Autodesk Inventor part; units mm, degrees
(part 2 of 6)
  line L517 (-101.2642, 134.6037) -> (-101.2642, 126.9657)
  line L518 (-101.2642, 126.9657) -> (-97.138, 126.9657)
  spline S136 degree 2 poles (-97.138, 126.9657) (-96.7341, 126.9657) (-96.1722, 126.4038) (-96.1722, 126) knots 0 0 0 1 2 2 2
  spline S137 degree 2 poles (-96.1722, 126) (-96.1722, 125.6137) (-96.7341, 125.0518) (-97.138, 125.0518) knots 0 0 0 1 2 2 2
  line L519 (-97.138, 125.0518) -> (-101.2642, 125.0518)
  line L520 (-101.2642, 125.0518) -> (-101.2642, 117.4139)
  line L521 (-101.2642, 117.4139) -> (-96.1547, 117.4139)
  spline S138 degree 2 poles (-96.1547, 117.4139) (-95.7684, 117.4139) (-95.2065, 116.852) (-95.2065, 116.4482) knots 0 0 0 1 2 2 2
  spline S139 degree 2 poles (-95.2065, 116.4482) (-95.2065, 116.0794) (-95.7684, 115.5) (-96.1547, 115.5) knots 0 0 0 1 2 2 2
  line L522 (-96.1547, 115.5) -> (-102.2299, 115.5)
  spline S140 degree 2 poles (-102.2299, 115.5) (-102.6162, 115.5) (-103.1781, 116.0619) (-103.1781, 116.4482) knots 0 0 0 1 2 2 2
  line L523 (-103.1781, 116.4482) -> (-103.1781, 135.5518)
  spline S141 degree 2 poles (-65.183, 124.1564) (-64.744, 124.2793) (-64.3577, 124.648) knots 0 0 0 1 1 1
  spline S142 degree 2 poles (-64.3577, 124.648) (-63.7958, 125.2099) (-63.7958, 126) knots 0 0 0 1 1 1
  line L524 (-63.7958, 126) -> (-63.7958, 132.6898)
  spline S143 degree 2 poles (-63.7958, 132.6898) (-63.7958, 133.4799) (-64.9196, 134.6037) (-65.7097, 134.6037) knots 0 0 0 1 2 2 2
  line L525 (-65.7097, 134.6037) -> (-68.8878, 134.6037)
  line L526 (-68.8878, 134.6037) -> (-68.8878, 116.4482)
  spline S144 degree 2 poles (-68.8878, 116.4482) (-68.8878, 116.0619) (-69.4497, 115.5) (-69.8535, 115.5) knots 0 0 0 1 2 2 2
  spline S145 degree 2 poles (-69.8535, 115.5) (-70.2398, 115.5) (-70.8017, 116.0619) (-70.8017, 116.4482) knots 0 0 0 1 2 2 2
  line L527 (-70.8017, 116.4482) -> (-70.8017, 135.5518)
  spline S146 degree 2 poles (-70.8017, 135.5518) (-70.8017, 135.9557) (-70.2398, 136.5) (-69.8535, 136.5) knots 0 0 0 1 2 2 2
  line L528 (-69.8535, 136.5) -> (-65.7097, 136.5)
  spline S147 degree 2 poles (-65.7097, 136.5) (-64.1295, 136.5) (-61.882, 134.2701) (-61.882, 132.6898) knots 0 0 0 1 2 2 2
  line L529 (-61.882, 132.6898) -> (-61.882, 126)
  spline S148 degree 2 poles (-61.882, 126) (-61.882, 124.4373) (-63.0057, 123.3135) knots 0 0 0 1 1 1
  spline S149 degree 2 poles (-63.0057, 123.3135) (-63.3569, 122.9624) (-63.7432, 122.7341) knots 0 0 0 1 1 1
  line L530 (-63.7432, 122.7341) -> (-61.3552, 116.8696)
  spline S150 degree 2 poles (-61.3552, 116.8696) (-61.2499, 116.6589) (-61.2499, 116.4482) knots 0 0 0 1 1 1
  spline S151 degree 2 poles (-61.2499, 116.4482) (-61.2499, 116.3077) (-61.3025, 116.1672) knots 0 0 0 1 1 1
  spline S152 degree 2 poles (-61.3025, 116.1672) (-61.4254, 115.7809) (-61.7766, 115.6054) knots 0 0 0 1 1 1
  spline S153 degree 2 poles (-61.7766, 115.6054) (-61.9873, 115.5) (-62.198, 115.5) knots 0 0 0 1 1 1
  spline S154 degree 2 poles (-62.198, 115.5) (-62.356, 115.5) (-62.4965, 115.5351) knots 0 0 0 1 1 1
  spline S155 degree 2 poles (-62.4965, 115.5351) (-62.8828, 115.658) (-63.0584, 116.0268) knots 0 0 0 1 1 1
  line L531 (-63.0584, 116.0268) -> (-65.78, 122.7692)
  spline S156 degree 2 poles (-65.78, 122.7692) (-65.9029, 122.9799) (-65.9029, 123.2433) knots 0 0 0 1 1 1
  spline S157 degree 2 poles (-65.9029, 123.2433) (-65.9029, 123.6296) (-65.6044, 123.9281) knots 0 0 0 1 1 1
  spline S158 degree 2 poles (-65.6044, 123.9281) (-65.4288, 124.1037) (-65.183, 124.1564) knots 0 0 0 1 1 1
  spline S159 degree 2 poles (-37.0031, 134.6037) (-37.3894, 134.6037) (-37.9512, 135.148) (-37.9512, 135.5518) knots 0 0 0 1 2 2 2
  spline S160 degree 2 poles (-37.9512, 135.5518) (-37.9512, 135.9557) (-37.3894, 136.5) (-37.0031, 136.5) knots 0 0 0 1 2 2 2
  line L532 (-37.0031, 136.5) -> (-29.9972, 136.5)
  spline S161 degree 2 poles (-29.9972, 136.5) (-29.5934, 136.5) (-29.0315, 135.9557) (-29.0315, 135.5518) knots 0 0 0 1 2 2 2
  spline S162 degree 2 poles (-29.0315, 135.5518) (-29.0315, 135.148) (-29.5934, 134.6037) (-29.9972, 134.6037) knots 0 0 0 1 2 2 2
  line L533 (-29.9972, 134.6037) -> (-32.5432, 134.6037)
  line L534 (-32.5432, 134.6037) -> (-32.5432, 116.4482)
  spline S163 degree 2 poles (-32.5432, 116.4482) (-32.5432, 116.0619) (-33.0875, 115.5) (-33.4914, 115.5) knots 0 0 0 1 2 2 2
  spline S164 degree 2 poles (-33.4914, 115.5) (-33.8952, 115.5) (-34.4571, 116.0619) (-34.4571, 116.4482) knots 0 0 0 1 2 2 2
  line L535 (-34.4571, 116.4482) -> (-34.4571, 134.6037)
  line L536 (-34.4571, 134.6037) -> (-37.0031, 134.6037)
  spline S165 degree 2 poles (-4.4511, 135.8503) (-4.4511, 136.2542) (-3.8892, 136.8161) (-3.5029, 136.8161) knots 0 0 0 1 2 2 2
  spline S166 degree 2 poles (-3.5029, 136.8161) (-3.0991, 136.8161) (-2.5372, 136.2542) (-2.5372, 135.8503) knots 0 0 0 1 2 2 2
  line L537 (-2.5372, 135.8503) -> (-2.5372, 119.9599)
  spline S167 degree 2 poles (-2.5372, 119.9599) (-2.5372, 118.9064) (-1.0447, 117.4139) (0.0088, 117.4139) knots 0 0 0 1 2 2 2
  spline S168 degree 2 poles (0.0088, 117.4139) (1.0623, 117.4139) (2.5548, 118.9064) (2.5548, 119.9599) knots 0 0 0 1 2 2 2
  line L538 (2.5548, 119.9599) -> (2.5548, 135.8503)
  spline S169 degree 2 poles (2.5548, 135.8503) (2.5548, 136.2542) (3.0991, 136.8161) (3.5029, 136.8161) knots 0 0 0 1 2 2 2
  spline S170 degree 2 poles (3.5029, 136.8161) (3.9068, 136.8161) (4.4686, 136.2542) (4.4686, 135.8503) knots 0 0 0 1 2 2 2
  line L539 (4.4686, 135.8503) -> (4.4686, 119.9599)
  spline S171 degree 2 poles (4.4686, 119.9599) (4.4686, 118.1162) (1.8524, 115.5) (0.0088, 115.5) knots 0 0 0 1 2 2 2
  spline S172 degree 2 poles (0.0088, 115.5) (-1.8349, 115.5) (-4.4511, 118.1162) (-4.4511, 119.9599) knots 0 0 0 1 2 2 2
  line L540 (-4.4511, 119.9599) -> (-4.4511, 135.8503)
  spline S173 degree 2 poles (38.118, 119.9423) (38.118, 118.0987) (36.8011, 116.7993) knots 0 0 0 1 1 1
  spline S174 degree 2 poles (36.8011, 116.7993) (35.6423, 115.6054) (34.0445, 115.5) knots 0 0 0 1 1 1
  spline S175 degree 2 poles (34.0445, 115.5) (33.5704, 115.5) (33.0261, 116.0619) (33.0261, 116.4482) knots 0 0 0 1 2 2 2
  spline S176 degree 2 poles (33.0261, 116.4482) (33.0261, 116.852) (33.307, 117.1329) knots 0 0 0 1 1 1
  spline S177 degree 2 poles (33.307, 117.1329) (33.5353, 117.3788) (33.8864, 117.4139) knots 0 0 0 1 1 1
  spline S178 degree 2 poles (33.8864, 117.4139) (34.7995, 117.4841) (35.4491, 118.1513) knots 0 0 0 1 1 1
  spline S179 degree 2 poles (35.4491, 118.1513) (36.2042, 118.8888) (36.2042, 119.9423) knots 0 0 0 1 1 1
  line L541 (36.2042, 119.9423) -> (36.2042, 122.5585)
  spline S180 degree 2 poles (36.2042, 122.5585) (36.2042, 123.5945) (35.4491, 124.3495) knots 0 0 0 1 1 1
  spline S181 degree 2 poles (35.4491, 124.3495) (34.8521, 124.964) (34.0445, 125.0694) knots 0 0 0 1 1 1
  spline S182 degree 2 poles (34.0445, 125.0694) (33.5704, 125.0694) (33.307, 125.3503) knots 0 0 0 1 1 1
  spline S183 degree 2 poles (33.307, 125.3503) (33.0261, 125.6313) (33.0261, 126.0176) knots 0 0 0 1 1 1
  line L542 (33.0261, 126.0176) -> (33.0261, 126.0351)
  spline S184 degree 2 poles (33.0261, 126.0351) (33.0261, 126.439) (33.307, 126.7199) knots 0 0 0 1 1 1
  spline S185 degree 2 poles (33.307, 126.7199) (33.5704, 127.0008) (34.0445, 127.0008) knots 0 0 0 1 1 1
  spline S186 degree 2 poles (34.0445, 127.0008) (34.8521, 127.1062) (35.4491, 127.7032) knots 0 0 0 1 1 1
  spline S187 degree 2 poles (35.4491, 127.7032) (36.2042, 128.4582) (36.2042, 129.5117) knots 0 0 0 1 1 1
  line L543 (36.2042, 129.5117) -> (36.2042, 132.0928)
  spline S188 degree 2 poles (36.2042, 132.0928) (36.2042, 133.1288) (35.4491, 133.8838) knots 0 0 0 1 1 1
  spline S189 degree 2 poles (35.4491, 133.8838) (34.7995, 134.5334) (33.8864, 134.6212) knots 0 0 0 1 1 1
  spline S190 degree 2 poles (33.8864, 134.6212) (33.5353, 134.6564) (33.307, 134.9022) knots 0 0 0 1 1 1
  spline S191 degree 2 poles (33.307, 134.9022) (33.0261, 135.1656) (33.0261, 135.5694) knots 0 0 0 1 1 1
  spline S192 degree 2 poles (33.0261, 135.5694) (33.0261, 135.9732) (33.5704, 136.5176) (34.0445, 136.5176) knots 0 0 0 1 2 2 2
  spline S193 degree 2 poles (34.0445, 136.5176) (35.6423, 136.4122) (36.8011, 135.2358) knots 0 0 0 1 1 1
  spline S194 degree 2 poles (36.8011, 135.2358) (38.118, 133.9365) (38.118, 132.0928) knots 0 0 0 1 1 1
  line L544 (38.118, 132.0928) -> (38.118, 129.5117)
  spline S195 degree 2 poles (38.118, 129.5117) (38.118, 127.3344) (36.45, 126.0176) knots 0 0 0 1 1 1
  spline S196 degree 2 poles (36.45, 126.0176) (38.118, 124.7182) (38.118, 122.5585) knots 0 0 0 1 1 1
  line L545 (38.118, 122.5585) -> (38.118, 119.9423)
  spline S197 degree 2 poles (29.1983, 135.5694) (29.1983, 135.9732) (29.7602, 136.5176) (30.1465, 136.5176) knots 0 0 0 1 2 2 2
  spline S198 degree 2 poles (30.1465, 136.5176) (30.5503, 136.5176) (31.1122, 135.9732) (31.1122, 135.5694) knots 0 0 0 1 2 2 2
  line L546 (31.1122, 135.5694) -> (31.1122, 116.4657)
  spline S199 degree 2 poles (31.1122, 116.4657) (31.1122, 116.0794) (30.5503, 115.5176) (30.1465, 115.5176) knots 0 0 0 1 2 2 2
  spline S200 degree 2 poles (30.1465, 115.5176) (29.7602, 115.5176) (29.1983, 116.0794) (29.1983, 116.4657) knots 0 0 0 1 2 2 2
  line L547 (29.1983, 116.4657) -> (29.1983, 135.5694)
  spline S201 degree 2 poles (69.8448, 126.9657) (70.2486, 126.9657) (70.8105, 126.4038) (70.8105, 126) knots 0 0 0 1 2 2 2
  spline S202 degree 2 poles (70.8105, 126) (70.8105, 125.6137) (70.2486, 125.0518) (69.8448, 125.0518) knots 0 0 0 1 2 2 2
  line L548 (69.8448, 125.0518) -> (65.7185, 125.0518)
  line L549 (65.7185, 125.0518) -> (65.7185, 116.4482)
  spline S203 degree 2 poles (65.7185, 116.4482) (65.7185, 116.0619) (65.1566, 115.5) (64.7528, 115.5) knots 0 0 0 1 2 2 2
  spline S204 degree 2 poles (64.7528, 115.5) (64.3665, 115.5) (63.8046, 116.0619) (63.8046, 116.4482) knots 0 0 0 1 2 2 2
  line L550 (63.8046, 116.4482) -> (63.8046, 135.5518)
  spline S205 degree 2 poles (63.8046, 135.5518) (63.8046, 135.9557) (64.3665, 136.5) (64.7528, 136.5) knots 0 0 0 1 2 2 2
  line L551 (64.7528, 136.5) -> (70.828, 136.5)
  spline S206 degree 2 poles (70.828, 136.5) (71.2143, 136.5) (71.7762, 135.9557) (71.7762, 135.5518) knots 0 0 0 1 2 2 2
  spline S207 degree 2 poles (71.7762, 135.5518) (71.7762, 135.1656) (71.2143, 134.6037) (70.828, 134.6037) knots 0 0 0 1 2 2 2
  line L552 (70.828, 134.6037) -> (65.7185, 134.6037)
  line L553 (65.7185, 134.6037) -> (65.7185, 126.9657)
  line L554 (65.7185, 126.9657) -> (69.8448, 126.9657)
  spline S208 degree 2 poles (96.2249, 134.6037) (95.8211, 134.6037) (95.2592, 135.148) (95.2592, 135.5518) knots 0 0 0 1 2 2 2
  spline S209 degree 2 poles (95.2592, 135.5518) (95.2592, 135.9557) (95.8211, 136.5) (96.2249, 136.5) knots 0 0 0 1 2 2 2
  line L555 (96.2249, 136.5) -> (103.5468, 136.5)
  spline S210 degree 2 poles (103.5468, 136.5) (103.9331, 136.5) (104.495, 135.9557) (104.495, 135.5518) knots 0 0 0 1 2 2 2
  spline S211 degree 2 poles (104.495, 135.5518) (104.495, 135.3587) (104.4247, 135.1831) knots 0 0 0 1 1 1
  line L556 (104.4247, 135.1831) -> (97.612, 117.4139)
  line L557 (97.612, 117.4139) -> (103.5468, 117.4139)
  spline S212 degree 2 poles (103.5468, 117.4139) (103.9331, 117.4139) (104.495, 116.852) (104.495, 116.4482) knots 0 0 0 1 2 2 2
  spline S213 degree 2 poles (104.495, 116.4482) (104.495, 116.0794) (103.9331, 115.5) (103.5468, 115.5) knots 0 0 0 1 2 2 2
  line L558 (103.5468, 115.5) -> (96.2249, 115.5)
  spline S214 degree 2 poles (96.2249, 115.5) (95.8386, 115.5) (95.2768, 116.0794) (95.2768, 116.4482) knots 0 0 0 1 2 2 2
  spline S215 degree 2 poles (95.2768, 116.4482) (95.2768, 116.694) (95.3645, 116.8871) knots 0 0 0 1 1 1
  line L559 (95.3645, 116.8871) -> (102.1421, 134.6037)
  line L560 (102.1421, 134.6037) -> (96.2249, 134.6037)
  spline S216 degree 2 poles (133.3421, 121.8211) (133.7284, 121.8211) (134.2903, 121.2592) (134.2903, 120.8554) knots 0 0 0 1 2 2 2
  spline S217 degree 2 poles (134.2903, 120.8554) (134.2903, 120.4691) (133.7284, 119.9072) (133.3421, 119.9072) knots 0 0 0 1 2 2 2
  line L561 (133.3421, 119.9072) -> (130.164, 119.9072)
  line L562 (130.164, 119.9072) -> (129.1983, 116.2901)
  spline S218 degree 2 poles (129.1983, 116.2901) (129.1105, 115.9916) (128.9174, 115.7809) knots 0 0 0 1 1 1
  spline S219 degree 2 poles (128.9174, 115.7809) (128.6364, 115.5) (128.2501, 115.5) knots 0 0 0 1 1 1
  spline S220 degree 2 poles (128.2501, 115.5) (127.8463, 115.5) (127.2844, 116.0619) (127.2844, 116.4482) knots 0 0 0 1 2 2 2
  spline S221 degree 2 poles (127.2844, 116.4482) (127.2844, 116.5711) (127.302, 116.6589) knots 0 0 0 1 1 1
  line L563 (127.302, 116.6589) -> (132.394, 135.6572)
  spline S222 degree 2 poles (132.394, 135.6572) (132.4642, 135.9732) (132.6749, 136.2015) knots 0 0 0 1 1 1
  spline S223 degree 2 poles (132.6749, 136.2015) (132.9558, 136.5) (133.3421, 136.5) knots 0 0 0 1 1 1
  spline S224 degree 2 poles (133.3421, 136.5) (133.7284, 136.5) (134.0269, 136.2015) knots 0 0 0 1 1 1
  spline S225 degree 2 poles (134.0269, 136.2015) (134.2025, 135.9732) (134.2727, 135.6572) knots 0 0 0 1 1 1
  line L564 (134.2727, 135.6572) -> (139.3647, 116.6589)
  spline S226 degree 2 poles (139.3647, 116.6589) (139.3822, 116.5711) (139.3822, 116.4482) knots 0 0 0 1 1 1
  spline S227 degree 2 poles (139.3822, 116.4482) (139.3822, 116.0619) (138.8204, 115.5) (138.4341, 115.5) knots 0 0 0 1 2 2 2
  spline S228 degree 2 poles (138.4341, 115.5) (138.0302, 115.5) (137.7669, 115.7809) knots 0 0 0 1 1 1
  spline S229 degree 2 poles (137.7669, 115.7809) (137.5562, 115.9916) (137.4684, 116.2901) knots 0 0 0 1 1 1
  line L565 (137.4684, 116.2901) -> (133.3421, 131.7943)
  line L566 (133.3421, 131.7943) -> (130.6732, 121.8211)
  line L567 (130.6732, 121.8211) -> (133.3421, 121.8211)
  spline S230 degree 2 poles (131.0244, 141.6095) (131.5511, 141.6095) (132.3062, 140.8545) (132.3062, 140.3278) knots 0 0 0 1 2 2 2
  spline S231 degree 2 poles (132.3062, 140.3278) (132.3062, 139.801) (131.5511, 139.0635) (131.0244, 139.0635) knots 0 0 0 1 2 2 2
  spline S232 degree 2 poles (131.0244, 139.0635) (130.4976, 139.0635) (129.7602, 139.801) (129.7602, 140.3278) knots 0 0 0 1 2 2 2
  spline S233 degree 2 poles (129.7602, 140.3278) (129.7602, 140.8545) (130.4976, 141.6095) (131.0244, 141.6095) knots 0 0 0 1 2 2 2
  spline S234 degree 2 poles (135.6598, 141.6095) (136.1866, 141.6095) (136.9241, 140.8545) (136.9241, 140.3278) knots 0 0 0 1 2 2 2
  spline S235 degree 2 poles (136.9241, 140.3278) (136.9241, 139.801) (136.1866, 139.0635) (135.6598, 139.0635) knots 0 0 0 1 2 2 2
  spline S236 degree 2 poles (135.6598, 139.0635) (135.1331, 139.0635) (134.3781, 139.801) (134.3781, 140.3278) knots 0 0 0 1 2 2 2
  spline S237 degree 2 poles (134.3781, 140.3278) (134.3781, 140.8545) (135.1331, 141.6095) (135.6598, 141.6095) knots 0 0 0 1 2 2 2
  spline S238 degree 2 poles (166.6754, 121.8211) (167.0617, 121.8211) (167.6236, 121.2592) (167.6236, 120.8554) knots 0 0 0 1 2 2 2
  spline S239 degree 2 poles (167.6236, 120.8554) (167.6236, 120.4691) (167.0617, 119.9072) (166.6754, 119.9072) knots 0 0 0 1 2 2 2
  line L568 (166.6754, 119.9072) -> (163.4974, 119.9072)
  line L569 (163.4974, 119.9072) -> (162.5316, 116.2901)
  spline S240 degree 2 poles (162.5316, 116.2901) (162.4438, 115.9916) (162.2507, 115.7809) knots 0 0 0 1 1 1
  spline S241 degree 2 poles (162.2507, 115.7809) (161.9698, 115.5) (161.5835, 115.5) knots 0 0 0 1 1 1
  spline S242 degree 2 poles (161.5835, 115.5) (161.1796, 115.5) (160.6178, 116.0619) (160.6178, 116.4482) knots 0 0 0 1 2 2 2
  spline S243 degree 2 poles (160.6178, 116.4482) (160.6178, 116.5711) (160.6353, 116.6589) knots 0 0 0 1 1 1
  line L570 (160.6353, 116.6589) -> (165.7273, 135.6572)
  spline S244 degree 2 poles (165.7273, 135.6572) (165.7975, 135.9732) (166.0082, 136.2015) knots 0 0 0 1 1 1
  spline S245 degree 2 poles (166.0082, 136.2015) (166.2892, 136.5) (166.6754, 136.5) knots 0 0 0 1 1 1
  spline S246 degree 2 poles (166.6754, 136.5) (167.0617, 136.5) (167.3602, 136.2015) knots 0 0 0 1 1 1
  spline S247 degree 2 poles (167.3602, 136.2015) (167.5358, 135.9732) (167.606, 135.6572) knots 0 0 0 1 1 1
  line L571 (167.606, 135.6572) -> (172.698, 116.6589)
  spline S248 degree 2 poles (172.698, 116.6589) (172.7156, 116.5711) (172.7156, 116.4482) knots 0 0 0 1 1 1
  spline S249 degree 2 poles (172.7156, 116.4482) (172.7156, 116.0619) (172.1537, 115.5) (171.7674, 115.5) knots 0 0 0 1 2 2 2
  spline S250 degree 2 poles (171.7674, 115.5) (171.3636, 115.5) (171.1002, 115.7809) knots 0 0 0 1 1 1
  spline S251 degree 2 poles (171.1002, 115.7809) (170.8895, 115.9916) (170.8017, 116.2901) knots 0 0 0 1 1 1
  line L572 (170.8017, 116.2901) -> (166.6754, 131.7943)
  line L573 (166.6754, 131.7943) -> (164.0065, 121.8211)
  line L574 (164.0065, 121.8211) -> (166.6754, 121.8211)
  spline S252 degree 2 poles (164.3577, 141.6095) (164.8845, 141.6095) (165.6395, 140.8545) (165.6395, 140.3278) knots 0 0 0 1 2 2 2
  spline S253 degree 2 poles (165.6395, 140.3278) (165.6395, 139.801) (164.8845, 139.0635) (164.3577, 139.0635) knots 0 0 0 1 2 2 2
  spline S254 degree 2 poles (164.3577, 139.0635) (163.831, 139.0635) (163.0935, 139.801) (163.0935, 140.3278) knots 0 0 0 1 2 2 2
  spline S255 degree 2 poles (163.0935, 140.3278) (163.0935, 140.8545) (163.831, 141.6095) (164.3577, 141.6095) knots 0 0 0 1 2 2 2
  spline S256 degree 2 poles (168.9932, 141.6095) (169.5199, 141.6095) (170.2574, 140.8545) (170.2574, 140.3278) knots 0 0 0 1 2 2 2
  spline S257 degree 2 poles (170.2574, 140.3278) (170.2574, 139.801) (169.5199, 139.0635) (168.9932, 139.0635) knots 0 0 0 1 2 2 2
  spline S258 degree 2 poles (168.9932, 139.0635) (168.4664, 139.0635) (167.7114, 139.801) (167.7114, 140.3278) knots 0 0 0 1 2 2 2
  spline S259 degree 2 poles (167.7114, 140.3278) (167.7114, 140.8545) (168.4664, 141.6095) (168.9932, 141.6095) knots 0 0 0 1 2 2 2
  spline S260 degree 2 poles (168.1504, 88.1564) (168.5893, 88.2793) (168.9756, 88.648) knots 0 0 0 1 1 1
  spline S261 degree 2 poles (168.9756, 88.648) (169.5375, 89.2099) (169.5375, 90) knots 0 0 0 1 1 1
  line L575 (169.5375, 90) -> (169.5375, 96.6898)
  spline S262 degree 2 poles (169.5375, 96.6898) (169.5375, 97.4799) (168.4137, 98.6037) (167.6236, 98.6037) knots 0 0 0 1 2 2 2
  line L576 (167.6236, 98.6037) -> (164.4455, 98.6037)
  line L577 (164.4455, 98.6037) -> (164.4455, 80.4482)
  spline S263 degree 2 poles (164.4455, 80.4482) (164.4455, 80.0619) (163.8836, 79.5) (163.4798, 79.5) knots 0 0 0 1 2 2 2
  spline S264 degree 2 poles (163.4798, 79.5) (163.0935, 79.5) (162.5316, 80.0619) (162.5316, 80.4482) knots 0 0 0 1 2 2 2
  line L578 (162.5316, 80.4482) -> (162.5316, 99.5518)
  spline S265 degree 2 poles (162.5316, 99.5518) (162.5316, 99.9557) (163.0935, 100.5) (163.4798, 100.5) knots 0 0 0 1 2 2 2
  line L579 (163.4798, 100.5) -> (167.6236, 100.5)
  spline S266 degree 2 poles (167.6236, 100.5) (169.2039, 100.5) (171.4514, 98.2701) (171.4514, 96.6898) knots 0 0 0 1 2 2 2
  line L580 (171.4514, 96.6898) -> (171.4514, 90)
  spline S267 degree 2 poles (171.4514, 90) (171.4514, 88.4373) (170.3276, 87.3135) knots 0 0 0 1 1 1
  spline S268 degree 2 poles (170.3276, 87.3135) (169.9764, 86.9624) (169.5902, 86.7341) knots 0 0 0 1 1 1
  line L581 (169.5902, 86.7341) -> (171.9781, 80.8696)
  spline S269 degree 2 poles (171.9781, 80.8696) (172.0835, 80.6589) (172.0835, 80.4482) knots 0 0 0 1 1 1
  spline S270 degree 2 poles (172.0835, 80.4482) (172.0835, 80.3077) (172.0308, 80.1672) knots 0 0 0 1 1 1
  spline S271 degree 2 poles (172.0308, 80.1672) (171.9079, 79.7809) (171.5567, 79.6054) knots 0 0 0 1 1 1
  spline S272 degree 2 poles (171.5567, 79.6054) (171.346, 79.5) (171.1353, 79.5) knots 0 0 0 1 1 1
  spline S273 degree 2 poles (171.1353, 79.5) (170.9773, 79.5) (170.8368, 79.5351) knots 0 0 0 1 1 1
  spline S274 degree 2 poles (170.8368, 79.5351) (170.4505, 79.658) (170.2749, 80.0268) knots 0 0 0 1 1 1
  line L582 (170.2749, 80.0268) -> (167.5534, 86.7692)
  spline S275 degree 2 poles (167.5534, 86.7692) (167.4305, 86.9799) (167.4305, 87.2433) knots 0 0 0 1 1 1
  spline S276 degree 2 poles (167.4305, 87.2433) (167.4305, 87.6296) (167.729, 87.9281) knots 0 0 0 1 1 1
  spline S277 degree 2 poles (167.729, 87.9281) (167.9045, 88.1037) (168.1504, 88.1564) knots 0 0 0 1 1 1
  spline S278 degree 2 poles (130.8664, 100.3595) (131.1122, 100.5176) (131.4282, 100.5176) knots 0 0 0 1 1 1
  spline S279 degree 2 poles (131.4282, 100.5176) (131.8145, 100.5176) (132.3764, 99.9557) (132.3764, 99.5694) knots 0 0 0 1 2 2 2
  spline S280 degree 2 poles (132.3764, 99.5694) (132.3764, 99.1656) (132.113, 98.9022) knots 0 0 0 1 1 1
  spline S281 degree 2 poles (132.113, 98.9022) (132.0252, 98.8319) (131.955, 98.7617) knots 0 0 0 1 1 1
  spline S282 degree 2 poles (131.955, 98.7617) (131.7267, 98.6212) (131.5336, 98.4281) knots 0 0 0 1 1 1
  spline S283 degree 2 poles (131.5336, 98.4281) (130.7961, 97.6731) (130.7961, 96.6196) knots 0 0 0 1 1 1
  line L583 (130.7961, 96.6196) -> (130.7961, 83.398)
  spline S284 degree 2 poles (130.7961, 83.398) (130.7961, 82.3445) (131.5336, 81.607) knots 0 0 0 1 1 1
  spline S285 degree 2 poles (131.5336, 81.607) (131.7267, 81.4139) (131.955, 81.2734) knots 0 0 0 1 1 1
  spline S286 degree 2 poles (131.955, 81.2734) (132.0252, 81.2207) (132.0955, 81.1505) knots 0 0 0 1 1 1
  spline S287 degree 2 poles (132.0955, 81.1505) (132.3764, 80.8696) (132.3764, 80.4657) knots 0 0 0 1 1 1
  spline S288 degree 2 poles (132.3764, 80.4657) (132.3764, 80.0794) (131.8145, 79.5176) (131.4282, 79.5176) knots 0 0 0 1 2 2 2
  spline S289 degree 2 poles (131.4282, 79.5176) (131.1297, 79.5176) (130.9015, 79.658) knots 0 0 0 1 1 1
  spline S290 degree 2 poles (130.9015, 79.658) (130.5152, 79.9214) (130.1816, 80.255) knots 0 0 0 1 1 1
  spline S291 degree 2 poles (130.1816, 80.255) (128.8822, 81.5543) (128.8822, 83.398) knots 0 0 0 1 1 1
  line L584 (128.8822, 83.398) -> (128.8822, 96.6196)
  spline S292 degree 2 poles (128.8822, 96.6196) (128.8822, 98.4808) (130.1816, 99.7801) knots 0 0 0 1 1 1
  spline S293 degree 2 poles (130.1816, 99.7801) (130.5152, 100.1137) (130.8664, 100.3595) knots 0 0 0 1 1 1
  spline S294 degree 2 poles (134.8346, 98.6915) (134.6941, 98.7617) (134.5712, 98.8846) knots 0 0 0 1 1 1
  spline S295 degree 2 poles (134.5712, 98.8846) (134.2903, 99.1656) (134.2903, 99.5518) knots 0 0 0 1 1 1
  spline S296 degree 2 poles (134.2903, 99.5518) (134.2903, 99.9557) (134.8521, 100.5176) (135.2384, 100.5176) knots 0 0 0 1 2 2 2
  spline S297 degree 2 poles (135.2384, 100.5176) (135.5545, 100.5176) (135.8179, 100.342) knots 0 0 0 1 1 1
  spline S298 degree 2 poles (135.8179, 100.342) (136.169, 100.0962) (136.4851, 99.7801) knots 0 0 0 1 1 1
  spline S299 degree 2 poles (136.4851, 99.7801) (137.7844, 98.4808) (137.7844, 96.6196) knots 0 0 0 1 1 1
  line L585 (137.7844, 96.6196) -> (137.7844, 83.398)
  spline S300 degree 2 poles (137.7844, 83.398) (137.7844, 81.5543) (136.4851, 80.255) knots 0 0 0 1 1 1
  spline S301 degree 2 poles (136.4851, 80.255) (136.1339, 79.9038) (135.7476, 79.6405) knots 0 0 0 1 1 1
  spline S302 degree 2 poles (135.7476, 79.6405) (135.5369, 79.5) (135.2384, 79.5) knots 0 0 0 1 1 1
  spline S303 degree 2 poles (135.2384, 79.5) (134.8521, 79.5) (134.2903, 80.0794) (134.2903, 80.4482) knots 0 0 0 1 2 2 2
  spline S304 degree 2 poles (134.2903, 80.4482) (134.2903, 80.852) (134.5712, 81.1329) knots 0 0 0 1 1 1
  spline S305 degree 2 poles (134.5712, 81.1329) (134.6414, 81.2032) (134.7117, 81.2559) knots 0 0 0 1 1 1
  spline S306 degree 2 poles (134.7117, 81.2559) (134.9224, 81.3963) (135.1331, 81.607) knots 0 0 0 1 1 1
  spline S307 degree 2 poles (135.1331, 81.607) (135.8881, 82.3445) (135.8881, 83.398) knots 0 0 0 1 1 1
  line L586 (135.8881, 83.398) -> (135.8881, 96.6196)
  spline S308 degree 2 poles (135.8881, 96.6196) (135.8881, 97.6731) (135.1331, 98.4281) knots 0 0 0 1 1 1
  spline S309 degree 2 poles (135.1331, 98.4281) (134.9926, 98.5686) (134.8346, 98.6915) knots 0 0 0 1 1 1
  spline S310 degree 2 poles (93.9686, 99.3411) (93.9511, 99.4465) (93.9511, 99.5518) knots 0 0 0 1 1 1
  spline S311 degree 2 poles (93.9511, 99.5518) (93.9511, 99.9557) (94.513, 100.5) (94.9168, 100.5) knots 0 0 0 1 2 2 2
  spline S312 degree 2 poles (94.9168, 100.5) (95.3031, 100.5) (95.584, 100.2366) knots 0 0 0 1 1 1
  spline S313 degree 2 poles (95.584, 100.2366) (95.7947, 100.0084) (95.865, 99.7099) knots 0 0 0 1 1 1
  line L587 (95.865, 99.7099) -> (100.0088, 84.1881)
  line L588 (100.0088, 84.1881) -> (104.135, 99.7099)
  spline S314 degree 2 poles (104.135, 99.7099) (104.2053, 100.0084) (104.4335, 100.2366) knots 0 0 0 1 1 1
  spline S315 degree 2 poles (104.4335, 100.2366) (104.6969, 100.5) (105.1008, 100.5) knots 0 0 0 1 1 1
  spline S316 degree 2 poles (105.1008, 100.5) (105.487, 100.5) (106.0489, 99.9557) (106.0489, 99.5518) knots 0 0 0 1 2 2 2
  spline S317 degree 2 poles (106.0489, 99.5518) (106.0489, 99.4465) (106.0314, 99.3411) knots 0 0 0 1 1 1
  line L589 (106.0314, 99.3411) -> (100.9394, 80.3253)
  spline S318 degree 2 poles (100.9394, 80.3253) (100.8691, 80.0268) (100.6936, 79.7809) knots 0 0 0 1 1 1
  spline S319 degree 2 poles (100.6936, 79.7809) (100.3951, 79.5) (100.0088, 79.5) knots 0 0 0 1 1 1
  spline S320 degree 2 poles (100.0088, 79.5) (99.6225, 79.5) (99.3416, 79.7809) knots 0 0 0 1 1 1
  spline S321 degree 2 poles (99.3416, 79.7809) (99.1309, 80.0268) (99.0606, 80.3253) knots 0 0 0 1 1 1
  line L590 (99.0606, 80.3253) -> (93.9686, 99.3411)
  spline S322 degree 2 poles (65.7097, 99.5518) (65.7097, 99.9557) (66.2716, 100.5) (66.6579, 100.5) knots 0 0 0 1 2 2 2
  spline S323 degree 2 poles (66.6579, 100.5) (67.0617, 100.5) (67.6236, 99.9557) (67.6236, 99.5518) knots 0 0 0 1 2 2 2
  line L591 (67.6236, 99.5518) -> (67.6236, 80.4482)
  spline S324 degree 2 poles (67.6236, 80.4482) (67.6236, 80.0619) (67.0617, 79.5) (66.6579, 79.5) knots 0 0 0 1 2 2 2
  spline S325 degree 2 poles (66.6579, 79.5) (66.2716, 79.5) (65.7097, 80.0619) (65.7097, 80.4482) knots 0 0 0 1 2 2 2
  line L592 (65.7097, 80.4482) -> (65.7097, 99.5518)
  spline S326 degree 2 poles (29.7865, 80.9749) (29.488, 81.3261) (29.488, 81.7299) knots 0 0 0 1 1 1
  spline S327 degree 2 poles (29.488, 81.7299) (29.5231, 82.1338) (29.8041, 82.3972) knots 0 0 0 1 1 1
  spline S328 degree 2 poles (29.8041, 82.3972) (30.0674, 82.643) (30.4889, 82.643) knots 0 0 0 1 1 1
  spline S329 degree 2 poles (30.4889, 82.643) (30.8751, 82.6079) (31.2088, 82.2742) knots 0 0 0 1 1 1
  spline S330 degree 2 poles (31.2088, 82.2742) (31.9111, 81.4841) (32.9646, 81.4314) knots 0 0 0 1 1 1
  line L593 (32.9646, 81.4314) -> (33.0875, 81.4314)
  spline S331 degree 2 poles (33.0875, 81.4314) (34.0708, 81.4314) (34.7907, 82.0987) knots 0 0 0 1 1 1
  spline S332 degree 2 poles (34.7907, 82.0987) (35.5808, 82.801) (35.6335, 83.837) knots 0 0 0 1 1 1
  line L594 (35.6335, 83.837) -> (35.6335, 84.0477)
  spline S333 degree 2 poles (35.6335, 84.0477) (35.6335, 86.6814) (32.4378, 90.2107) knots 0 0 0 1 1 1
  spline S334 degree 2 poles (32.4378, 90.2107) (29.2598, 93.7224) (29.2598, 96.6722) knots 0 0 0 1 1 1
  line L595 (29.2598, 96.6722) -> (29.2598, 96.9356)
  spline S335 degree 2 poles (29.2598, 96.9356) (29.3651, 98.7968) (30.7347, 100.0259) knots 0 0 0 1 1 1
  spline S336 degree 2 poles (30.7347, 100.0259) (32.0164, 101.1672) (33.6845, 101.1672) knots 0 0 0 1 1 1
  line L596 (33.6845, 101.1672) -> (33.9479, 101.1672)
  spline S337 degree 2 poles (33.9479, 101.1672) (35.8091, 101.0619) (37.0206, 99.6923) knots 0 0 0 1 1 1
  spline S338 degree 2 poles (37.0206, 99.6923) (37.3367, 99.3411) (37.3367, 98.9548) knots 0 0 0 1 1 1
  spline S339 degree 2 poles (37.3367, 98.9548) (37.3016, 98.551) (37.0031, 98.2876) knots 0 0 0 1 1 1
  spline S340 degree 2 poles (37.0031, 98.2876) (36.7397, 98.0418) (36.371, 98.0418) knots 0 0 0 1 1 1
  spline S341 degree 2 poles (36.371, 98.0418) (35.932, 98.0594) (35.6335, 98.4105) knots 0 0 0 1 1 1
  spline S342 degree 2 poles (35.6335, 98.4105) (34.896, 99.1831) (33.8425, 99.2358) knots 0 0 0 1 1 1
  line L597 (33.8425, 99.2358) -> (33.6669, 99.2358)
  spline S343 degree 2 poles (33.6669, 99.2358) (32.7363, 99.2358) (32.0164, 98.6037) knots 0 0 0 1 1 1
  spline S344 degree 2 poles (32.0164, 98.6037) (31.2263, 97.8838) (31.1736, 96.8303) knots 0 0 0 1 1 1
  line L598 (31.1736, 96.8303) -> (31.1736, 96.6898)
  spline S345 degree 2 poles (31.1736, 96.6898) (31.1736, 94.4774) (34.4044, 90.9306) knots 0 0 0 1 1 1
  spline S346 degree 2 poles (34.4044, 90.9306) (37.5649, 87.4189) (37.5649, 84.1003) knots 0 0 0 1 1 1
  spline S347 degree 2 poles (37.5649, 84.1003) (37.5649, 83.9247) (37.5474, 83.7492) knots 0 0 0 1 1 1
  spline S348 degree 2 poles (37.5474, 83.7492) (37.442, 81.888) (36.0725, 80.6413) knots 0 0 0 1 1 1
  spline S349 degree 2 poles (36.0725, 80.6413) (34.7907, 79.5) (33.1051, 79.5) knots 0 0 0 1 1 1
  line L599 (33.1051, 79.5) -> (32.8593, 79.5)
  spline S350 degree 2 poles (32.8593, 79.5) (31.0156, 79.6054) (29.7865, 80.9749) knots 0 0 0 1 1 1
  spline S351 degree 2 poles (3.1957, 99.4816) (3.459, 99.1831) (3.459, 98.8144) knots 0 0 0 1 1 1
  spline S352 degree 2 poles (3.459, 98.8144) (3.459, 98.4105) (2.8972, 97.8487) (2.5109, 97.8487) knots 0 0 0 1 2 2 2
  spline S353 degree 2 poles (2.5109, 97.8487) (2.107, 97.8487) (1.8436, 98.1296) knots 0 0 0 1 1 1
  spline S354 degree 2 poles (1.8436, 98.1296) (1.036, 98.9197) (0, 98.9197) knots 0 0 0 1 1 1
  spline S355 degree 2 poles (0, 98.9197) (-1.0711, 98.9197) (-2.546, 97.4273) (-2.546, 96.3737) knots 0 0 0 1 2 2 2
  line L600 (-2.546, 96.3737) -> (-2.546, 83.9599)
  spline S356 degree 2 poles (-2.546, 83.9599) (-2.546, 82.9064) (-1.0711, 81.4139) (0, 81.4139) knots 0 0 0 1 2 2 2
  line L601 (0, 81.4139) -> (2.546, 81.4139)
  line L602 (2.546, 81.4139) -> (2.546, 88.7358)
  line L603 (2.546, 88.7358) -> (1.5803, 88.7358)
  spline S357 degree 2 poles (1.5803, 88.7358) (1.194, 88.7358) (0.6321, 89.2977) (0.6321, 89.6839) knots 0 0 0 1 2 2 2
  spline S358 degree 2 poles (0.6321, 89.6839) (0.6321, 90.0878) (1.194, 90.6497) (1.5803, 90.6497) knots 0 0 0 1 2 2 2
  line L604 (1.5803, 90.6497) -> (3.5117, 90.6497)
  spline S359 degree 2 poles (3.5117, 90.6497) (3.9156, 90.6497) (4.4423, 90.0878) (4.4423, 89.6839) knots 0 0 0 1 2 2 2
  line L605 (4.4423, 89.6839) -> (4.4423, 80.4482)
  spline S360 degree 2 poles (4.4423, 80.4482) (4.4423, 80.0794) (3.898, 79.5) (3.4941, 79.5) knots 0 0 0 1 2 2 2
  line L606 (3.4941, 79.5) -> (0, 79.5)
  spline S361 degree 2 poles (0, 79.5) (-1.8612, 79.5) (-4.4599, 82.0987) (-4.4599, 83.9423) knots 0 0 0 1 2 2 2
  line L607 (-4.4599, 83.9423) -> (-4.4599, 96.3913)
  spline S362 degree 2 poles (-4.4599, 96.3913) (-4.4599, 98.2349) (-1.8612, 100.8512) (0, 100.8512) knots 0 0 0 1 2 2 2
  spline S363 degree 2 poles (0, 100.8512) (1.8436, 100.8512) (3.1957, 99.4816) knots 0 0 0 1 1 1
  spline S364 degree 2 poles (-37.1084, 98.6037) (-37.5123, 98.6037) (-38.0741, 99.148) (-38.0741, 99.5518) knots 0 0 0 1 2 2 2
  spline S365 degree 2 poles (-38.0741, 99.5518) (-38.0741, 99.9557) (-37.5123, 100.5) (-37.1084, 100.5) knots 0 0 0 1 2 2 2
  line L608 (-37.1084, 100.5) -> (-29.7865, 100.5)
  spline S366 degree 2 poles (-29.7865, 100.5) (-29.4002, 100.5) (-28.8384, 99.9557) (-28.8384, 99.5518) knots 0 0 0 1 2 2 2
  spline S367 degree 2 poles (-28.8384, 99.5518) (-28.8384, 99.3587) (-28.9086, 99.1831) knots 0 0 0 1 1 1
  line L609 (-28.9086, 99.1831) -> (-35.7213, 81.4139)
  line L610 (-35.7213, 81.4139) -> (-29.7865, 81.4139)
  spline S368 degree 2 poles (-29.7865, 81.4139) (-29.4002, 81.4139) (-28.8384, 80.852) (-28.8384, 80.4482) knots 0 0 0 1 2 2 2
  spline S369 degree 2 poles (-28.8384, 80.4482) (-28.8384, 80.0794) (-29.4002, 79.5) (-29.7865, 79.5) knots 0 0 0 1 2 2 2
  line L611 (-29.7865, 79.5) -> (-37.1084, 79.5)
  spline S370 degree 2 poles (-37.1084, 79.5) (-37.4947, 79.5) (-38.0566, 80.0794) (-38.0566, 80.4482) knots 0 0 0 1 2 2 2
  spline S371 degree 2 poles (-38.0566, 80.4482) (-38.0566, 80.694) (-37.9688, 80.8871) knots 0 0 0 1 1 1
  line L612 (-37.9688, 80.8871) -> (-31.1912, 98.6037)
  line L613 (-31.1912, 98.6037) -> (-37.1084, 98.6037)
  spline S372 degree 2 poles (-70.1608, 80.4482) (-70.1608, 80.0619) (-70.7227, 79.5) (-71.1265, 79.5) knots 0 0 0 1 2 2 2
  spline S373 degree 2 poles (-71.1265, 79.5) (-71.5128, 79.5) (-72.0747, 80.0619) (-72.0747, 80.4482) knots 0 0 0 1 2 2 2
  line L614 (-72.0747, 80.4482) -> (-72.0747, 99.5694)
  spline S374 degree 2 poles (-72.0747, 99.5694) (-72.0747, 99.9732) (-71.5128, 100.5176) (-71.1265, 100.5176) knots 0 0 0 1 2 2 2
  spline S375 degree 2 poles (-71.1265, 100.5176) (-70.7227, 100.5176) (-70.4417, 100.2542) knots 0 0 0 1 1 1
  spline S376 degree 2 poles (-70.4417, 100.2542) (-70.3364, 100.1488) (-70.2837, 100.0259) knots 0 0 0 1 1 1
  line L615 (-70.2837, 100.0259) -> (-63.155, 84.7324)
  line L616 (-63.155, 84.7324) -> (-63.155, 99.5694)
  spline S377 degree 2 poles (-63.155, 99.5694) (-63.155, 99.9732) (-62.6106, 100.5176) (-62.2068, 100.5176) knots 0 0 0 1 2 2 2
  spline S378 degree 2 poles (-62.2068, 100.5176) (-61.803, 100.5176) (-61.2586, 99.9732) (-61.2586, 99.5694) knots 0 0 0 1 2 2 2
  line L617 (-61.2586, 99.5694) -> (-61.2586, 80.4306)
  spline S379 degree 2 poles (-61.2586, 80.4306) (-61.2586, 80.0619) (-61.522, 79.7809) knots 0 0 0 1 1 1
  spline S380 degree 2 poles (-61.522, 79.7809) (-61.803, 79.5) (-62.2068, 79.5) knots 0 0 0 1 1 1
  spline S381 degree 2 poles (-62.2068, 79.5) (-62.6106, 79.5) (-62.874, 79.7809) knots 0 0 0 1 1 1
  spline S382 degree 2 poles (-62.874, 79.7809) (-63.0145, 79.9214) (-63.1198, 80.1321) knots 0 0 0 1 1 1
  line L618 (-63.1198, 80.1321) -> (-70.1608, 95.3729)
  line L619 (-70.1608, 95.3729) -> (-70.1608, 80.4482)
  spline S383 degree 2 poles (-99.9912, 85.8211) (-99.6049, 85.8211) (-99.0431, 85.2592) (-99.0431, 84.8554) knots 0 0 0 1 2 2 2
  spline S384 degree 2 poles (-99.0431, 84.8554) (-99.0431, 84.4691) (-99.6049, 83.9072) (-99.9912, 83.9072) knots 0 0 0 1 2 2 2
  line L620 (-99.9912, 83.9072) -> (-103.1693, 83.9072)
  line L621 (-103.1693, 83.9072) -> (-104.135, 80.2901)
  spline S385 degree 2 poles (-104.135, 80.2901) (-104.2228, 79.9916) (-104.416, 79.7809) knots 0 0 0 1 1 1
  spline S386 degree 2 poles (-104.416, 79.7809) (-104.6969, 79.5) (-105.0832, 79.5) knots 0 0 0 1 1 1
  spline S387 degree 2 poles (-105.0832, 79.5) (-105.487, 79.5) (-106.0489, 80.0619) (-106.0489, 80.4482) knots 0 0 0 1 2 2 2
  spline S388 degree 2 poles (-106.0489, 80.4482) (-106.0489, 80.5711) (-106.0314, 80.6589) knots 0 0 0 1 1 1
  line L622 (-106.0314, 80.6589) -> (-100.9394, 99.6572)
  spline S389 degree 2 poles (-100.9394, 99.6572) (-100.8691, 99.9732) (-100.6584, 100.2015) knots 0 0 0 1 1 1
  spline S390 degree 2 poles (-100.6584, 100.2015) (-100.3775, 100.5) (-99.9912, 100.5) knots 0 0 0 1 1 1
  spline S391 degree 2 poles (-99.9912, 100.5) (-99.6049, 100.5) (-99.3064, 100.2015) knots 0 0 0 1 1 1
  spline S392 degree 2 poles (-99.3064, 100.2015) (-99.1309, 99.9732) (-99.0606, 99.6572) knots 0 0 0 1 1 1
  line L623 (-99.0606, 99.6572) -> (-93.9686, 80.6589)
  spline S393 degree 2 poles (-93.9686, 80.6589) (-93.9511, 80.5711) (-93.9511, 80.4482) knots 0 0 0 1 1 1
  spline S394 degree 2 poles (-93.9511, 80.4482) (-93.9511, 80.0619) (-94.513, 79.5) (-94.8992, 79.5) knots 0 0 0 1 2 2 2
  spline S395 degree 2 poles (-94.8992, 79.5) (-95.3031, 79.5) (-95.5665, 79.7809) knots 0 0 0 1 1 1
  spline S396 degree 2 poles (-95.5665, 79.7809) (-95.7772, 79.9916) (-95.865, 80.2901) knots 0 0 0 1 1 1
  line L624 (-95.865, 80.2901) -> (-99.9912, 95.7943)
  line L625 (-99.9912, 95.7943) -> (-102.6601, 85.8211)
  line L626 (-102.6601, 85.8211) -> (-99.9912, 85.8211)
  spline S397 degree 2 poles (-102.3089, 105.6095) (-101.7822, 105.6095) (-101.0272, 104.8545) (-101.0272, 104.3278) knots 0 0 0 1 2 2 2
  spline S398 degree 2 poles (-101.0272, 104.3278) (-101.0272, 103.801) (-101.7822, 103.0635) (-102.3089, 103.0635) knots 0 0 0 1 2 2 2
  spline S399 degree 2 poles (-102.3089, 103.0635) (-102.8357, 103.0635) (-103.5732, 103.801) (-103.5732, 104.3278) knots 0 0 0 1 2 2 2
  spline S400 degree 2 poles (-103.5732, 104.3278) (-103.5732, 104.8545) (-102.8357, 105.6095) (-102.3089, 105.6095) knots 0 0 0 1 2 2 2
  spline S401 degree 2 poles (-97.6735, 105.6095) (-97.1467, 105.6095) (-96.4093, 104.8545) (-96.4093, 104.3278) knots 0 0 0 1 2 2 2
  spline S402 degree 2 poles (-96.4093, 104.3278) (-96.4093, 103.801) (-97.1467, 103.0635) (-97.6735, 103.0635) knots 0 0 0 1 2 2 2
  spline S403 degree 2 poles (-97.6735, 103.0635) (-98.2003, 103.0635) (-98.9553, 103.801) (-98.9553, 104.3278) knots 0 0 0 1 2 2 2
  spline S404 degree 2 poles (-98.9553, 104.3278) (-98.9553, 104.8545) (-98.2003, 105.6095) (-97.6735, 105.6095) knots 0 0 0 1 2 2 2
  spline S405 degree 2 poles (-128.496, 80.3253) (-128.5486, 80.0268) (-128.7769, 79.7809) knots 0 0 0 1 1 1
  spline S406 degree 2 poles (-128.7769, 79.7809) (-129.0578, 79.5) (-129.4441, 79.5) knots 0 0 0 1 1 1
  spline S407 degree 2 poles (-129.4441, 79.5) (-129.848, 79.5) (-130.1113, 79.7809) knots 0 0 0 1 1 1
  spline S408 degree 2 poles (-130.1113, 79.7809) (-130.322, 80.0268) (-130.3747, 80.3253) knots 0 0 0 1 1 1
  line L627 (-130.3747, 80.3253) -> (-133.3421, 92.3528)
  line L628 (-133.3421, 92.3528) -> (-136.2919, 80.3428)
  spline S409 degree 2 poles (-136.2919, 80.3428) (-136.3446, 80.0268) (-136.5729, 79.7809) knots 0 0 0 1 1 1
  spline S410 degree 2 poles (-136.5729, 79.7809) (-136.8538, 79.5) (-137.2401, 79.5) knots 0 0 0 1 1 1
  spline S411 degree 2 poles (-137.2401, 79.5) (-137.644, 79.5) (-137.9073, 79.7809) knots 0 0 0 1 1 1
  spline S412 degree 2 poles (-137.9073, 79.7809) (-138.1356, 80.0268) (-138.2058, 80.3253) knots 0 0 0 1 1 1
  line L629 (-138.2058, 80.3253) -> (-142.7886, 99.3411)
  spline S413 degree 2 poles (-142.7886, 99.3411) (-142.8062, 99.4465) (-142.8062, 99.5518) knots 0 0 0 1 1 1
  spline S414 degree 2 poles (-142.8062, 99.5518) (-142.8062, 99.9557) (-142.2618, 100.5) (-141.858, 100.5) knots 0 0 0 1 2 2 2
  spline S415 degree 2 poles (-141.858, 100.5) (-141.4542, 100.5) (-141.1732, 100.2366) knots 0 0 0 1 1 1
  spline S416 degree 2 poles (-141.1732, 100.2366) (-140.9625, 100.0084) (-140.9098, 99.7099) knots 0 0 0 1 1 1
  line L630 (-140.9098, 99.7099) -> (-137.2401, 84.5393)
  line L631 (-137.2401, 84.5393) -> (-134.3605, 96.3737)
  spline S417 degree 2 poles (-134.3605, 96.3737) (-134.2552, 96.8127) (-133.7284, 97.3219) (-133.3246, 97.3219) knots 0 0 0 1 2 2 2
  spline S418 degree 2 poles (-133.3246, 97.3219) (-132.9207, 97.3219) (-132.4115, 96.7776) (-132.3237, 96.3737) knots 0 0 0 1 2 2 2
  line L632 (-132.3237, 96.3737) -> (-129.4441, 84.5393)
  line L633 (-129.4441, 84.5393) -> (-125.7744, 99.7099)
  spline S419 degree 2 poles (-125.7744, 99.7099) (-125.7217, 100.0084) (-125.4935, 100.2366) knots 0 0 0 1 1 1
  spline S420 degree 2 poles (-125.4935, 100.2366) (-125.2301, 100.5) (-124.8262, 100.5) knots 0 0 0 1 1 1
  spline S421 degree 2 poles (-124.8262, 100.5) (-124.4224, 100.5) (-123.8781, 99.9557) (-123.8781, 99.5518) knots 0 0 0 1 2 2 2
  spline S422 degree 2 poles (-123.8781, 99.5518) (-123.8781, 99.4465) (-123.8956, 99.3411) knots 0 0 0 1 1 1
  line L634 (-123.8956, 99.3411) -> (-128.496, 80.3253)
  spline S423 degree 2 poles (-170.4417, 98.6037) (-170.8456, 98.6037) (-171.4075, 99.148) (-171.4075, 99.5518) knots 0 0 0 1 2 2 2
  spline S424 degree 2 poles (-171.4075, 99.5518) (-171.4075, 99.9557) (-170.8456, 100.5) (-170.4417, 100.5) knots 0 0 0 1 2 2 2
  line L635 (-170.4417, 100.5) -> (-163.1198, 100.5)
  spline S425 degree 2 poles (-163.1198, 100.5) (-162.7336, 100.5) (-162.1717, 99.9557) (-162.1717, 99.5518) knots 0 0 0 1 2 2 2
  spline S426 degree 2 poles (-162.1717, 99.5518) (-162.1717, 99.3587) (-162.2419, 99.1831) knots 0 0 0 1 1 1
  line L636 (-162.2419, 99.1831) -> (-169.0546, 81.4139)
  line L637 (-169.0546, 81.4139) -> (-163.1198, 81.4139)
  spline S427 degree 2 poles (-163.1198, 81.4139) (-162.7336, 81.4139) (-162.1717, 80.852) (-162.1717, 80.4482) knots 0 0 0 1 2 2 2
  spline S428 degree 2 poles (-162.1717, 80.4482) (-162.1717, 80.0794) (-162.7336, 79.5) (-163.1198, 79.5) knots 0 0 0 1 2 2 2
  line L638 (-163.1198, 79.5) -> (-170.4417, 79.5)
  spline S429 degree 2 poles (-170.4417, 79.5) (-170.828, 79.5) (-171.3899, 80.0794) (-171.3899, 80.4482) knots 0 0 0 1 2 2 2
  spline S430 degree 2 poles (-171.3899, 80.4482) (-171.3899, 80.694) (-171.3021, 80.8871) knots 0 0 0 1 1 1
  line L639 (-171.3021, 80.8871) -> (-164.5245, 98.6037)
  line L640 (-164.5245, 98.6037) -> (-170.4417, 98.6037)
  spline S431 degree 2 poles (-166.6579, 49.8211) (-166.2716, 49.8211) (-165.7097, 49.2592) (-165.7097, 48.8554) knots 0 0 0 1 2 2 2
  spline S432 degree 2 poles (-165.7097, 48.8554) (-165.7097, 48.4691) (-166.2716, 47.9072) (-166.6579, 47.9072) knots 0 0 0 1 2 2 2
  line L641 (-166.6579, 47.9072) -> (-169.836, 47.9072)
  line L642 (-169.836, 47.9072) -> (-170.8017, 44.2901)
  spline S433 degree 2 poles (-170.8017, 44.2901) (-170.8895, 43.9916) (-171.0826, 43.7809) knots 0 0 0 1 1 1
  spline S434 degree 2 poles (-171.0826, 43.7809) (-171.3636, 43.5) (-171.7499, 43.5) knots 0 0 0 1 1 1
  spline S435 degree 2 poles (-171.7499, 43.5) (-172.1537, 43.5) (-172.7156, 44.0619) (-172.7156, 44.4482) knots 0 0 0 1 2 2 2
  spline S436 degree 2 poles (-172.7156, 44.4482) (-172.7156, 44.5711) (-172.698, 44.6589) knots 0 0 0 1 1 1
  line L643 (-172.698, 44.6589) -> (-167.606, 63.6572)
  spline S437 degree 2 poles (-167.606, 63.6572) (-167.5358, 63.9732) (-167.3251, 64.2015) knots 0 0 0 1 1 1
  spline S438 degree 2 poles (-167.3251, 64.2015) (-167.0442, 64.5) (-166.6579, 64.5) knots 0 0 0 1 1 1
  spline S439 degree 2 poles (-166.6579, 64.5) (-166.2716, 64.5) (-165.9731, 64.2015) knots 0 0 0 1 1 1
  spline S440 degree 2 poles (-165.9731, 64.2015) (-165.7975, 63.9732) (-165.7273, 63.6572) knots 0 0 0 1 1 1
  line L644 (-165.7273, 63.6572) -> (-160.6353, 44.6589)
  spline S441 degree 2 poles (-160.6353, 44.6589) (-160.6178, 44.5711) (-160.6178, 44.4482) knots 0 0 0 1 1 1
  spline S442 degree 2 poles (-160.6178, 44.4482) (-160.6178, 44.0619) (-161.1796, 43.5) (-161.5659, 43.5) knots 0 0 0 1 2 2 2
  spline S443 degree 2 poles (-161.5659, 43.5) (-161.9698, 43.5) (-162.2331, 43.7809) knots 0 0 0 1 1 1
  spline S444 degree 2 poles (-162.2331, 43.7809) (-162.4438, 43.9916) (-162.5316, 44.2901) knots 0 0 0 1 1 1
  line L645 (-162.5316, 44.2901) -> (-166.6579, 59.7943)
  line L646 (-166.6579, 59.7943) -> (-169.3268, 49.8211)
  line L647 (-169.3268, 49.8211) -> (-166.6579, 49.8211)
  spline S445 degree 2 poles (-128.5486, 47.9423) (-128.5486, 46.0987) (-129.8655, 44.7993) knots 0 0 0 1 1 1
  spline S446 degree 2 poles (-129.8655, 44.7993) (-131.0244, 43.6054) (-132.6222, 43.5) knots 0 0 0 1 1 1
  spline S447 degree 2 poles (-132.6222, 43.5) (-133.0963, 43.5) (-133.6406, 44.0619) (-133.6406, 44.4482) knots 0 0 0 1 2 2 2
  spline S448 degree 2 poles (-133.6406, 44.4482) (-133.6406, 44.852) (-133.3597, 45.1329) knots 0 0 0 1 1 1
  spline S449 degree 2 poles (-133.3597, 45.1329) (-133.1314, 45.3788) (-132.7802, 45.4139) knots 0 0 0 1 1 1
  spline S450 degree 2 poles (-132.7802, 45.4139) (-131.8672, 45.4841) (-131.2175, 46.1513) knots 0 0 0 1 1 1
  spline S451 degree 2 poles (-131.2175, 46.1513) (-130.4625, 46.8888) (-130.4625, 47.9423) knots 0 0 0 1 1 1
  line L648 (-130.4625, 47.9423) -> (-130.4625, 50.5585)
  spline S452 degree 2 poles (-130.4625, 50.5585) (-130.4625, 51.5945) (-131.2175, 52.3495) knots 0 0 0 1 1 1
  spline S453 degree 2 poles (-131.2175, 52.3495) (-131.8145, 52.964) (-132.6222, 53.0694) knots 0 0 0 1 1 1
  spline S454 degree 2 poles (-132.6222, 53.0694) (-133.0963, 53.0694) (-133.3597, 53.3503) knots 0 0 0 1 1 1
  spline S455 degree 2 poles (-133.3597, 53.3503) (-133.6406, 53.6313) (-133.6406, 54.0176) knots 0 0 0 1 1 1
  line L649 (-133.6406, 54.0176) -> (-133.6406, 54.0351)
  spline S456 degree 2 poles (-133.6406, 54.0351) (-133.6406, 54.439) (-133.3597, 54.7199) knots 0 0 0 1 1 1
  spline S457 degree 2 poles (-133.3597, 54.7199) (-133.0963, 55.0008) (-132.6222, 55.0008) knots 0 0 0 1 1 1
  spline S458 degree 2 poles (-132.6222, 55.0008) (-131.8145, 55.1062) (-131.2175, 55.7032) knots 0 0 0 1 1 1
  spline S459 degree 2 poles (-131.2175, 55.7032) (-130.4625, 56.4582) (-130.4625, 57.5117) knots 0 0 0 1 1 1
  line L650 (-130.4625, 57.5117) -> (-130.4625, 60.0928)
  spline S460 degree 2 poles (-130.4625, 60.0928) (-130.4625, 61.1288) (-131.2175, 61.8838) knots 0 0 0 1 1 1
  spline S461 degree 2 poles (-131.2175, 61.8838) (-131.8672, 62.5334) (-132.7802, 62.6212) knots 0 0 0 1 1 1
  spline S462 degree 2 poles (-132.7802, 62.6212) (-133.1314, 62.6564) (-133.3597, 62.9022) knots 0 0 0 1 1 1
  spline S463 degree 2 poles (-133.3597, 62.9022) (-133.6406, 63.1656) (-133.6406, 63.5694) knots 0 0 0 1 1 1
  spline S464 degree 2 poles (-133.6406, 63.5694) (-133.6406, 63.9732) (-133.0963, 64.5176) (-132.6222, 64.5176) knots 0 0 0 1 2 2 2
  spline S465 degree 2 poles (-132.6222, 64.5176) (-131.0244, 64.4122) (-129.8655, 63.2358) knots 0 0 0 1 1 1
  spline S466 degree 2 poles (-129.8655, 63.2358) (-128.5486, 61.9365) (-128.5486, 60.0928) knots 0 0 0 1 1 1
  line L651 (-128.5486, 60.0928) -> (-128.5486, 57.5117)
  spline S467 degree 2 poles (-128.5486, 57.5117) (-128.5486, 55.3344) (-130.2167, 54.0176) knots 0 0 0 1 1 1
  spline S468 degree 2 poles (-130.2167, 54.0176) (-128.5486, 52.7182) (-128.5486, 50.5585) knots 0 0 0 1 1 1
  line L652 (-128.5486, 50.5585) -> (-128.5486, 47.9423)
  spline S469 degree 2 poles (-137.4684, 63.5694) (-137.4684, 63.9732) (-136.9065, 64.5176) (-136.5202, 64.5176) knots 0 0 0 1 2 2 2
  spline S470 degree 2 poles (-136.5202, 64.5176) (-136.1164, 64.5176) (-135.5545, 63.9732) (-135.5545, 63.5694) knots 0 0 0 1 2 2 2
  line L653 (-135.5545, 63.5694) -> (-135.5545, 44.4657)
  spline S471 degree 2 poles (-135.5545, 44.4657) (-135.5545, 44.0794) (-136.1164, 43.5176) (-136.5202, 43.5176) knots 0 0 0 1 2 2 2
  spline S472 degree 2 poles (-136.5202, 43.5176) (-136.9065, 43.5176) (-137.4684, 44.0794) (-137.4684, 44.4657) knots 0 0 0 1 2 2 2
  line L654 (-137.4684, 44.4657) -> (-137.4684, 63.5694)
  spline S473 degree 2 poles (-102.467, 64.3595) (-102.2212, 64.5176) (-101.9051, 64.5176) knots 0 0 0 1 1 1
  spline S474 degree 2 poles (-101.9051, 64.5176) (-101.5188, 64.5176) (-100.9569, 63.9557) (-100.9569, 63.5694) knots 0 0 0 1 2 2 2
  spline S475 degree 2 poles (-100.9569, 63.5694) (-100.9569, 63.1656) (-101.2203, 62.9022) knots 0 0 0 1 1 1
  spline S476 degree 2 poles (-101.2203, 62.9022) (-101.3081, 62.8319) (-101.3783, 62.7617) knots 0 0 0 1 1 1
  spline S477 degree 2 poles (-101.3783, 62.7617) (-101.6066, 62.6212) (-101.7997, 62.4281) knots 0 0 0 1 1 1
  spline S478 degree 2 poles (-101.7997, 62.4281) (-102.5372, 61.6731) (-102.5372, 60.6196) knots 0 0 0 1 1 1
  line L655 (-102.5372, 60.6196) -> (-102.5372, 47.398)
  spline S479 degree 2 poles (-102.5372, 47.398) (-102.5372, 46.3445) (-101.7997, 45.607) knots 0 0 0 1 1 1
  spline S480 degree 2 poles (-101.7997, 45.607) (-101.6066, 45.4139) (-101.3783, 45.2734) knots 0 0 0 1 1 1
  spline S481 degree 2 poles (-101.3783, 45.2734) (-101.3081, 45.2207) (-101.2379, 45.1505) knots 0 0 0 1 1 1
  spline S482 degree 2 poles (-101.2379, 45.1505) (-100.9569, 44.8696) (-100.9569, 44.4657) knots 0 0 0 1 1 1
  spline S483 degree 2 poles (-100.9569, 44.4657) (-100.9569, 44.0794) (-101.5188, 43.5176) (-101.9051, 43.5176) knots 0 0 0 1 2 2 2
  spline S484 degree 2 poles (-101.9051, 43.5176) (-102.2036, 43.5176) (-102.4319, 43.658) knots 0 0 0 1 1 1
  spline S485 degree 2 poles (-102.4319, 43.658) (-102.8181, 43.9214) (-103.1518, 44.255) knots 0 0 0 1 1 1
  spline S486 degree 2 poles (-103.1518, 44.255) (-104.4511, 45.5543) (-104.4511, 47.398) knots 0 0 0 1 1 1
  line L656 (-104.4511, 47.398) -> (-104.4511, 60.6196)
  spline S487 degree 2 poles (-104.4511, 60.6196) (-104.4511, 62.4808) (-103.1518, 63.7801) knots 0 0 0 1 1 1
  spline S488 degree 2 poles (-103.1518, 63.7801) (-102.8181, 64.1137) (-102.467, 64.3595) knots 0 0 0 1 1 1
  spline S489 degree 2 poles (-98.4987, 62.6915) (-98.6392, 62.7617) (-98.7621, 62.8846) knots 0 0 0 1 1 1
  spline S490 degree 2 poles (-98.7621, 62.8846) (-99.0431, 63.1656) (-99.0431, 63.5518) knots 0 0 0 1 1 1
  spline S491 degree 2 poles (-99.0431, 63.5518) (-99.0431, 63.9557) (-98.4812, 64.5176) (-98.0949, 64.5176) knots 0 0 0 1 2 2 2
  spline S492 degree 2 poles (-98.0949, 64.5176) (-97.7788, 64.5176) (-97.5155, 64.342) knots 0 0 0 1 1 1
  spline S493 degree 2 poles (-97.5155, 64.342) (-97.1643, 64.0962) (-96.8482, 63.7801) knots 0 0 0 1 1 1
  spline S494 degree 2 poles (-96.8482, 63.7801) (-95.5489, 62.4808) (-95.5489, 60.6196) knots 0 0 0 1 1 1
  line L657 (-95.5489, 60.6196) -> (-95.5489, 47.398)
  spline S495 degree 2 poles (-95.5489, 47.398) (-95.5489, 45.5543) (-96.8482, 44.255) knots 0 0 0 1 1 1
  spline S496 degree 2 poles (-96.8482, 44.255) (-97.1994, 43.9038) (-97.5857, 43.6405) knots 0 0 0 1 1 1
  spline S497 degree 2 poles (-97.5857, 43.6405) (-97.7964, 43.5) (-98.0949, 43.5) knots 0 0 0 1 1 1
  spline S498 degree 2 poles (-98.0949, 43.5) (-98.4812, 43.5) (-99.0431, 44.0794) (-99.0431, 44.4482) knots 0 0 0 1 2 2 2
  spline S499 degree 2 poles (-99.0431, 44.4482) (-99.0431, 44.852) (-98.7621, 45.1329) knots 0 0 0 1 1 1
  spline S500 degree 2 poles (-98.7621, 45.1329) (-98.6919, 45.2032) (-98.6217, 45.2559) knots 0 0 0 1 1 1
  spline S501 degree 2 poles (-98.6217, 45.2559) (-98.411, 45.3963) (-98.2003, 45.607) knots 0 0 0 1 1 1
  spline S502 degree 2 poles (-98.2003, 45.607) (-97.4452, 46.3445) (-97.4452, 47.398) knots 0 0 0 1 1 1
  line L658 (-97.4452, 47.398) -> (-97.4452, 60.6196)
  spline S503 degree 2 poles (-97.4452, 60.6196) (-97.4452, 61.6731) (-98.2003, 62.4281) knots 0 0 0 1 1 1